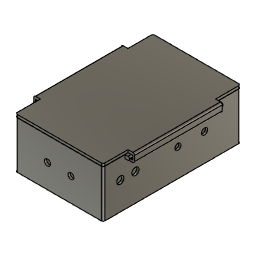
candlestick-mic (Autodesk Fusion 360 design; units mm, degrees)
Autodesk Fusion 360 part; units mm, degrees
note: some values were not read from the file. Set by a fixed rule: which sketch regions a step uses.
sketch "top" plane through (0, 0, 0) normal (0, 0, 1) x (1, 0, 0)
  line L0 (45.5, -15.075) -> (-45.5, -15.075) construction
  line L1 (-45.5, -15.075) -> (-45.5, 15.075) construction
  line L2 (-45.5, 15.075) -> (45.5, 15.075) construction
  line L3 (45.5, 15.075) -> (45.5, -15.075) construction
  line L4 (45.5, -15.075) -> (-45.5, 15.075) construction
  line L5 (-45.5, -15.075) -> (45.5, 15.075) construction
  line L6 (0, 15.075) -> (0, -15.075) construction
  line L7 (-45.5, 0) -> (45.5, 0) construction
  circle A0 centre (-40.35, 0) radius 2.1 construction
  line L8 (-35.35, 15.075) -> (-35.35, -15.075) construction
  circle A1 centre (40.35, 0) radius 2.1 construction
  line L9 (35.35, 15.075) -> (35.35, -15.075) construction
  line L10 (35.35, 33.075) -> (-4.8, 33.075) construction
  line L11 (-4.8, 33.075) -> (-4.8, 93.375) construction
  line L12 (-4.8, 93.375) -> (35.35, 93.375) construction
  line L13 (35.35, 93.375) -> (35.35, 33.075) construction
  line L14 (-45.5, 21.075) -> (-25.4, 21.075)
  line L15 (-25.4, 21.075) -> (-25.4, 101.225)
  line L16 (-25.4, 101.225) -> (-45.5, 101.225)
  line L17 (-45.5, 101.225) -> (-45.5, 21.075)
  line L18 (-4.8, 63.225) -> (35.35, 63.225) construction
  line L19 (15.275, 93.375) -> (15.275, 33.075) construction
  line L20 (-45.5, 61.15) -> (-25.4, 61.15) construction
  line L21 (-35.45, 101.225) -> (-35.45, 21.075) construction
  circle A2 centre (33.25, 35.175) radius 0.85
  circle A3 centre (33.25, 35.175) radius 2.35
  circle A4 centre (33.25, 91.275) radius 0.85
  circle A5 centre (33.25, 91.275) radius 2.35
  circle A6 centre (-2.7, 35.175) radius 0.85
  circle A7 centre (-2.7, 35.175) radius 2.35
  circle A8 centre (-2.7, 91.275) radius 2.35
  circle A9 centre (-2.7, 91.275) radius 0.85
  circle A10 centre (-27.5, 23.225) radius 0.85
  circle A11 centre (-27.5, 23.225) radius 2.1
  circle A12 centre (-27.5, 99.075) radius 0.85
  circle A13 centre (-27.5, 99.075) radius 2.1
  circle A14 centre (-43.4, 23.225) radius 0.85
  circle A15 centre (-43.4, 23.225) radius 2.1
  circle A16 centre (-43.4, 99.075) radius 0.85
  circle A17 centre (-43.4, 99.075) radius 2.1
  line L22 (-47.5, 101.725) -> (47.5, 101.725)
  line L23 (47.5, 101.725) -> (47.5, -50.075)
  line L24 (47.5, -50.075) -> (-47.5, -50.075)
  line L25 (-47.5, -50.075) -> (-47.5, 101.725)
  line L26 (-39.75, 101.225) -> (-29.75, 101.225)
  line L27 (-29.75, 101.225) -> (-29.75, 102.475)
  line L28 (-29.75, 102.475) -> (-39.75, 102.475)
  line L29 (-39.75, 102.475) -> (-39.75, 101.225)
  line L30 (-34.75, 102.475) -> (-34.75, 101.225) construction
  circle A18 centre (-40.35, 0) radius 1.75
  circle A19 centre (40.35, 0) radius 1.75
  line L31 (-50, -52.575) -> (-50, 104.225)
  line L32 (-50, 104.225) -> (50, 104.225)
  line L33 (50, 104.225) -> (50, -52.575)
  line L34 (50, -52.575) -> (-50, -52.575)
  circle A20 centre (-42.5, 76.725) radius 2.5
  dimension "d1" = 91
  dimension "d2" = 30.15
  dimension "d3" = 4.2
  dimension "d4" = 10.15
  dimension "d5" = 3.05
  dimension "d6" = 40.15
  dimension "d7" = 60.3
  dimension "d8" = 18
  dimension "d9" = 20.1
  dimension "d10" = 80.15
  dimension "d11" = 6
  dimension "d12" = 1.7
  dimension "d13" = 1.25
  dimension "d14" = 1.25
  dimension "d15" = 1.5
  dimension "d16" = 1.7
  dimension "d17" = 1.25
  dimension "d18" = 1.3
  dimension "d19" = 1.25
  dimension "d20" = 2
  dimension "d21" = 1.25
  dimension "d22" = 10
  dimension "d23" = 0.5
  dimension "d24" = 2
  dimension "d25" = 35
  dimension "d35" = -0.35
  dimension "d39" = -2.5
  dimension "d43" = 4.35
  dimension "d61" = 5
  dimension "d62" = 22
  dimension "d63" = 0.5
  constraint horizontal L0
  constraint perpendicular L0 L1
  constraint parallel L0 L2
  constraint parallel L1 L3
  constraint coincident L4 origin
  constraint coincident L5 origin
  constraint midpoint L2 L6.start
  constraint midpoint L0 L6.end
  constraint midpoint L1 L7.start
  constraint midpoint L3 L7.end
  constraint coincident L7 A0.centre
  constraint coincident L2 L8.start
  constraint coincident L0 L8.end
  constraint perpendicular L0 L8
  constraint symmetric L6 A0 A1
  constraint symmetric L6 L8.start L9.start
  constraint symmetric L6 L8.end L9.end
  constraint horizontal L10
  constraint vertical L11
  constraint horizontal L12
  constraint vertical L13
  constraint horizontal L14
  constraint vertical L15
  constraint horizontal L16
  constraint vertical L17
  constraint collinear L1 L17
  constraint collinear L9 L13
  constraint midpoint L11 L18.start
  constraint midpoint L13 L18.end
  constraint midpoint L12 L19.start
  constraint midpoint L10 L19.end
  constraint midpoint L17 L20.start
  constraint midpoint L15 L20.end
  constraint midpoint L16 L21.start
  constraint midpoint L14 L21.end
  constraint symmetric L18 A2 A4
  constraint symmetric L18 A3 A5
  constraint symmetric L19 A2 A6
  constraint symmetric L19 A3 A7
  constraint symmetric L19 A4 A9
  constraint symmetric L19 A5 A8
  constraint symmetric L20 A10 A12
  constraint symmetric L20 A11 A13
  constraint symmetric L21 A10 A14
  constraint symmetric L21 A11 A15
  constraint symmetric L21 A12 A16
  constraint symmetric L21 A13 A17
  constraint horizontal L22
  constraint vertical L23
  constraint horizontal L24
  constraint vertical L25
  constraint horizontal L26
  constraint vertical L27
  constraint horizontal L28
  constraint vertical L29
  constraint coincident L16 L26.start
  constraint midpoint L28 L30.start
  constraint midpoint L26 L30.end
  constraint symmetric L6 A18 A19
  measures "d1" distance of L1.end L2.end
  measures "d2" distance of L0.end L1.end
  measures "d3" diameter of A0
  measures "d4" distance of L1 L8
  measures "d5" distance of L1 A0
  measures "d6" distance of L10.start L10.end
  measures "d7" distance of L10.start L12.end
  measures "d8" distance of L2 L10
  measures "d9" distance of L14.start L14.end
  measures "d10" distance of L14.start L16.end
  measures "d11" distance of L2 L14
  measures "d12" diameter of A2
  measures "d13" distance of L13 A2
  measures "d14" distance of L10 A2
  measures "d16" diameter of A10
  measures "d17" distance of L15 A10
  measures "d18" distance of L14 A10
  measures "d20" distance of L17 L25
  measures "d21" distance of L26.end L27.end
  measures "d22" distance of L27.end L28.end
  measures "d23" distance of L16 L22
  measures "d24" distance of L3 L23
  measures "d25" distance of L0 L24
  measures "d43" distance of L15 L27
  measures "d61" diameter of A20
  measures "d62" distance of L16 A20
  measures "d63" distance of L17 A20
extrude "Extrude1" add sketch "top" along normal blind 9 contours A11 | A13 | A17 | A15 | L14 L15 L16 L17 L26 | L14 L15 L16 L17 L22 L23 L24 L25 L27 L29 | L16 L22 L26 L27 L29 | L22 L27 L28 L29 | A2 | A3 | A4 | A5 | A6 | A7 | A8 | A9 | A10 | A12 | A14 | A16 | A18 | A19 | L31 L32 L33 L34 | A20 makes body 1
extrude "Extrude2" add sketch "top" along normal blind 12 from surface at 9 contours A11 | A13 | A17 | A15 | A3 | A5 | A7 | A8 bodies 1
extrude "Extrude4" cut sketch "top" against normal blind 6.5 from surface at 9 contours A18 | A19 bodies 1
extrude "Extrude5" add sketch "top" along normal blind 45 from surface at 9 contours L22 L27 L28 L29 | L31 L32 L33 L34 bodies 1
sketch "outputs" plane through (47.5, 0, 0) normal (-1, 0, 0) x (0, -1, 0)
  line L0 (-101.725, 9) -> (50.075, 9)
  line L1 (50.075, 9) -> (50.075, 54)
  line L2 (50.075, 54) -> (-101.725, 54)
  line L3 (-101.725, 54) -> (-101.725, 9)
  line L4 (-32.825, 21) -> (-37.525, 21)
  line L5 (-88.925, 21) -> (-93.625, 21)
  line L6 (-93.625, 21) -> (-93.625, 54) construction
  line L7 (-32.825, 21) -> (-32.825, 54) construction
  line L8 (-93.625, 54) -> (-32.825, 54) construction
  line L9 (-88.925, 21) -> (-37.525, 21) construction
  line L10 (-63.225, 21) -> (-63.225, 54) construction
  circle A0 centre (-63.225, 31.5) radius 3.5
  circle A1 centre (-32.825, 31.5) radius 3.5
  line L11 (50.075, 31.5) -> (-32.825, 31.5) construction
  line L12 (25.825, 24.9389) -> (25.825, 54) construction
  circle A2 centre (32.95, 31.5) radius 4.125
  circle A3 centre (15.7, 31.5) radius 4.125
  line L13 (-32.825, 31.5) -> (-63.225, 31.5) construction
  dimension "d44" = 7
  dimension "d45" = 7
  dimension "d46" = 8.25
  dimension "d47" = 8.25
  dimension "d48" = 6
  dimension "d49" = 3
  dimension "d50" = 13
  constraint coincident L5.end L6.start
  constraint coincident L2 L6.end
  constraint perpendicular L2 L6
  constraint coincident L4.start L7.start
  constraint coincident L2 L7.end
  constraint perpendicular L2 L7
  constraint coincident L5.start L9.start
  constraint coincident L4.end L9.end
  constraint midpoint L9 L10.start
  constraint midpoint L8 L10.end
  constraint midpoint L1 L11.start
  constraint coincident L7 A1.centre
  constraint perpendicular L7 L11
  constraint coincident L2 L12.end
  constraint perpendicular L2 L12
  constraint coincident L11 A2.centre
  constraint coincident L11 A3.centre
  constraint coincident A1.centre L11.end
  constraint coincident L10 A0.centre
  constraint perpendicular L10 L13
  constraint coincident A0.centre L13.end
  measures "d44" diameter of A0
  measures "d45" diameter of A1
  measures "d46" diameter of A2
  measures "d47" diameter of A3
  measures "d48" distance of L12 A3
  measures "d49" distance of L12 A2
  measures "d50" distance of L1 A2
extrude "Extrude6" cut sketch "outputs" against normal blind 4 contours A0 | A1 | A2 | A3 bodies 1
extrude "Extrude7" add sketch "top" along normal blind 1.5 from surface at 21 separate body contours A11 | A13 | A17 | A15 | L14 L15 L16 L17 L26 | A10 | A12 | A14 | A16 | A20 makes body 2
extrude "Extrude8" add sketch "top" along normal blind 12 from surface at 22.5 contours L16 L22 L26 L27 L29 | L22 L27 L28 L29 bodies 2
extrude "Extrude9" cut 1 faces at (-33.0833, 102.475, 26.5) along direction (0, 1, 0) blind 5 on bodies 2 bodies 1
extrude "Extrude10" add sketch "top" along normal blind 7 from surface at 22.5 contours A20 bodies 2
sketch "side" plane through (-47.5, 0, 0) normal (1, 0, 0) x (0, 1, 0)
  line L0 (-50.075, 9) -> (101.725, 9)
  line L1 (101.725, 9) -> (101.725, 54)
  line L2 (101.725, 54) -> (-50.075, 54)
  line L3 (-50.075, 54) -> (-50.075, 9)
  line L4 (79.225, 29.5) -> (74.225, 29.5)
  line L5 (74.225, 22.5) -> (79.225, 22.5)
  line L6 (76.725, 29.5) -> (76.725, 22.5) construction
  line L7 (74.225, 29.5) -> (74.225, 22.5) construction
  line L8 (79.225, 29.5) -> (79.225, 22.5) construction
  line L9 (74.225, 26) -> (79.225, 26) construction
  line L10 (74.975, 27.75) -> (78.475, 27.75)
  line L11 (78.475, 27.75) -> (78.475, 24.25)
  line L12 (78.475, 24.25) -> (74.975, 24.25)
  line L13 (74.975, 24.25) -> (74.975, 27.75)
  line L14 (74.975, 26) -> (78.475, 26) construction
  line L15 (76.725, 27.75) -> (76.725, 24.25) construction
  point P0 (76.725, 26)
  point P1 (76.725, 26)
  dimension "d67" = 3.5
  dimension "d68" = 3.5
  constraint midpoint L4 L6.start
  constraint midpoint L5 L6.end
  constraint coincident L4.end L7.start
  constraint coincident L5.start L7.end
  constraint coincident L4.start L8.start
  constraint coincident L5.end L8.end
  constraint midpoint L7 L9.start
  constraint midpoint L8 L9.end
  constraint horizontal L10
  constraint vertical L11
  constraint horizontal L12
  constraint vertical L13
  constraint midpoint L6 P1
  constraint midpoint L13 L14.start
  constraint midpoint L11 L14.end
  constraint midpoint L10 L15.start
  constraint midpoint L12 L15.end
  constraint midpoint L14 P1
  constraint coincident P1 P0
  measures "d67" distance of L10.start L10.end
  measures "d68" distance of L10.start L12.end
extrude "Extrude11" cut sketch "side" against normal blind 5 contours L10 L11 L12 L13 bodies 1
extrude "Extrude12" cut 1 faces at (-33.0833, 102.475, 26.5) along direction (0, -1, 0) blind 1 on bodies 1 bodies 1
sketch "inputs" plane through (0, -52.575, 0) normal (0, -1, 0) x (1, 0, 0)
  line L0 (-50, 0) -> (50, 0)
  line L1 (50, 0) -> (50, 54)
  line L2 (50, 54) -> (-50, 54)
  line L3 (-50, 54) -> (-50, 0)
  line L4 (47.5, 9) -> (-47.5, 9)
  line L5 (-47.5, 9) -> (-47.5, 54)
  line L6 (-47.5, 54) -> (47.5, 54)
  line L7 (47.5, 54) -> (47.5, 9)
  line L8 (0, 54) -> (0, 9) construction
  line L9 (47.5, 31.5) -> (-47.5, 31.5) construction
  circle A0 centre (13.375, 27) radius 3.375
  circle A1 centre (-13.5, 27) radius 3.5
  line L10 (50, 0) -> (-50, 0)
  line L11 (-35.6219, 54) -> (-35.6219, 0) construction
  line L12 (-35.6219, 27) -> (47.5, 27) construction
  dimension "d73" = 6.75
  dimension "d74" = 7
  dimension "d75" = 10
  dimension "d76" = 10
  constraint midpoint L6 L8.start
  constraint midpoint L4 L8.end
  constraint midpoint L7 L9.start
  constraint midpoint L5 L9.end
  constraint coincident L2 L11.start
  constraint coincident L10 L11.end
  constraint perpendicular L10 L11
  constraint midpoint L11 L12.start
  constraint coincident L7 L12.end
  constraint perpendicular L7 L12
  constraint coincident A1.centre L12
  constraint coincident A0.centre L12
  measures "d73" diameter of A0
  measures "d74" diameter of A1
  measures "d75" distance of L8 A0
  measures "d76" distance of L8 A1
extrude "Extrude13" cut sketch "inputs" against normal blind 4 contours A0 | A1 bodies 1
sketch "lid_bottom" plane through (-50, 0, 0) normal (-1, 0, 0) x (0, -1, 0)
  line L0 (-78.475, 24.25) -> (-78.475, 27.75)
  line L1 (-78.475, 27.75) -> (-74.975, 27.75)
  line L2 (-74.975, 27.75) -> (-74.975, 24.25)
  line L3 (-74.975, 24.25) -> (-78.475, 24.25)
  line L4 (-104.225, 0) -> (52.575, 0)
  line L5 (52.575, 0) -> (52.575, 54)
  line L6 (52.575, 54) -> (-104.225, 54)
  line L7 (-104.225, 54) -> (-104.225, 0)
  line L8 (-104.225, 54) -> (52.575, 54)
  line L9 (-104.225, 0) -> (-104.225, 54)
  line L10 (52.575, 0) -> (-104.225, 0)
  line L11 (52.575, 0) -> (52.575, 54)
  line L12 (-25.825, 54) -> (-25.825, 0) construction
  line L13 (-25.825, 50) -> (27.575, 50)
  line L14 (27.575, 50) -> (27.575, 54)
  line L15 (-25.825, 50) -> (-79.225, 50)
  line L16 (-79.225, 50) -> (-79.225, 54)
  dimension "d79" = 25
  dimension "d80" = 4
  constraint midpoint L8 L12.start
  constraint midpoint L10 L12.end
  constraint coincident L12 L13.start
  constraint perpendicular L12 L13
  constraint coincident L8 L14.end
  constraint perpendicular L8 L14
  constraint symmetric L12 L13.start L15.start
  constraint symmetric L12 L13.end L15.end
  constraint symmetric L12 L14.end L16.end
  measures "d79" distance of L11 L14
  measures "d80" distance of L8 L13
extrude "Extrude14" add sketch "lid_bottom" along normal blind 5 contours L6 L8 L13 L14 L15 L16 bodies 1
extrude "Extrude15" add sketch "lid_bottom" against normal blind 5 from surface at -100 contours L6 L8 L13 L14 L15 L16 bodies 1
fillet "Fillet1" radius 1.5 4 edges at (-55, 25.825, 54) (-55, 25.825, 50) (55, 25.825, 54) (55, 25.825, 50) on bodies 1
sketch "lid_top" plane through (0, 104.225, 0) normal (0, 1, 0) x (-1, 0, 0)
  line L0 (29.75, 22.5) -> (29.75, 34.5)
  line L1 (29.75, 34.5) -> (39.75, 34.5)
  line L2 (39.75, 34.5) -> (39.75, 22.5)
  line L3 (39.75, 22.5) -> (29.75, 22.5)
  line L4 (-50, 0) -> (50, 0)
  line L5 (50, 0) -> (50, 54)
  line L6 (50, 54) -> (-50, 54)
  line L7 (-50, 54) -> (-50, 0)
  line L8 (50, 54) -> (53.5, 54)
  arc A0 (55, 52.5) -> (53.5, 54) centre (53.5, 52.5) ccw
  line L9 (55, 52.5) -> (55, 51.5)
  arc A1 (53.5, 50) -> (55, 51.5) centre (53.5, 51.5) ccw
  line L10 (50, 50) -> (53.5, 50)
  line L11 (50, 50) -> (50, 54)
  line L12 (-50, 54) -> (-53.5, 54)
  arc A2 (-53.5, 54) -> (-55, 52.5) centre (-53.5, 52.5) ccw
  arc A3 (-55, 51.5) -> (-53.5, 50) centre (-53.5, 51.5) ccw
  line L13 (-50, 50) -> (-53.5, 50)
  line L14 (-50, 54) -> (-50, 50)
  line L15 (-55, 51.5) -> (-55, 52.5)
  line L16 (-50, 54) -> (50, 54)
  line L17 (-55, 52) -> (-57.5, 52) construction
  line L18 (-51, 49.75) -> (-51, 47.25)
  line L19 (-57.5, 52) -> (-57.5, 57.25)
  line L20 (-57.5, 52) -> (-57.5, 47.25)
  line L21 (-57.5, 47.25) -> (-51, 47.25)
  line L22 (0, 54) -> (0, 70) construction
  line L23 (0, 54) -> (0, 39) construction
  line L24 (-55, 49.75) -> (-55, 54.25)
  line L25 (-57.5, 57.25) -> (0, 57.25)
  line L26 (-55, 54.25) -> (0, 54.25)
  line L27 (-55, 49.75) -> (-51, 49.75)
  line L28 (57.5, 57.25) -> (0, 57.25)
  line L29 (55, 54.25) -> (0, 54.25)
  line L30 (57.5, 52) -> (57.5, 57.25)
  line L31 (55, 49.75) -> (55, 54.25)
  line L32 (57.5, 52) -> (57.5, 47.25)
  line L33 (57.5, 47.25) -> (51, 47.25)
  line L34 (51, 49.75) -> (51, 47.25)
  line L35 (55, 49.75) -> (51, 49.75)
  line L36 (50, 57.25) -> (50, 54.25)
  line L37 (-50, 57.25) -> (-50, 54.25)
  line L38 (45.5, 21) -> (41.3, 21)
  line L39 (29.6, 21) -> (25.4, 21)
  line L40 (5.05, 21) -> (0.35, 21)
  line L41 (-30.9, 21) -> (-35.6, 21)
  line L42 (5.05, 21) -> (25.4, 21) construction
  line L43 (39.75, 22.5) -> (39.75, 34.5)
  line L44 (39.75, 34.5) -> (29.75, 34.5)
  line L45 (29.75, 34.5) -> (29.75, 22.5)
  line L46 (29.75, 22.5) -> (39.75, 22.5)
  line L47 (29.75, 28.5) -> (0, 28.5) construction
  line L48 (15.225, 21) -> (15.225, 28.5) construction
  circle A4 centre (15.225, 28.5) radius 3
  dimension "d88" = 2.5
  dimension "d90" = 2.5
  dimension "d91" = 2.5
  dimension "d92" = 1
  dimension "d94" = 0.25
  dimension "d95" = 3
  dimension "d96" = 4.5
  dimension "d108" = 7.5
  dimension "d119" = 6
  constraint midpoint L15 L17.start
  constraint perpendicular L15 L17
  constraint perpendicular L13 L18
  constraint perpendicular L17 L19
  constraint perpendicular L17 L20
  constraint perpendicular L20 L21
  constraint midpoint L6 L22.start
  constraint perpendicular L16 L22
  constraint perpendicular L16 L23
  constraint perpendicular L17 L24
  constraint coincident L22 L25.end
  constraint perpendicular L22 L25
  constraint coincident L22 L26.end
  constraint perpendicular L22 L26
  constraint perpendicular L18 L27
  constraint symmetric L17.end L23 L30.start
  constraint symmetric L18.start L23 L34.start
  constraint symmetric L18.end L23 L33.end
  constraint symmetric L19.end L23 L28.start
  constraint symmetric L20.end L23 L32.end
  constraint symmetric L23 L24.start L31.start
  constraint symmetric L23 L25.end L28.end
  constraint symmetric L23 L24.end L29.start
  constraint symmetric L23 L26.end L29.end
  constraint coincident L28 L36.start
  constraint coincident L29 L36.end
  constraint perpendicular L29 L36
  constraint symmetric L22 L36.start L37.start
  constraint symmetric L22 L36.end L37.end
  constraint coincident L40.start L42.start
  constraint coincident L39.end L42.end
  constraint midpoint L45 L47.start
  constraint perpendicular L45 L47
  constraint midpoint L42 L48.start
  constraint coincident L47 L48.end
  constraint perpendicular L47 L48
  constraint coincident L48.end A4.centre
  measures "d88" distance of L17.start L17.end
  measures "d90" distance of L18.start L18.end
  measures "d91" distance of L19 L24
  measures "d92" distance of L7 L18
  measures "d94" distance of L16 L26
  measures "d95" distance of L25 L26
  measures "d96" distance of L24.start L24.end
  measures "d108" distance of L30 L36
  measures "d119" diameter of A4
ref_plane "WorkPlane1" through (0, 25.825, 27) normal (0, -1, 0) x (1, 0, 0)
extrude "Extrude17" add sketch "lid_top" along normal blind 50 and the other way blind 50 from surface at -78.4 separate body contours L15 L18 L19 L20 L21 L24 L25 L26 L27 L37 | L9 L28 L29 L30 L31 L32 L33 L34 L35 L36 | L25 L26 L28 L29 L36 L37 makes body 3
extrude "Extrude18" add sketch "lid_top" against normal up to surface (28.4 mm away) from surface at -128.4 contours L25 L26 L28 L29 L36 L37 bodies 3
extrude "Extrude19" add sketch "lid_top" along normal up to surface (28.4 mm away) from surface at -28.4 contours L25 L26 L28 L29 L36 L37 bodies 3
fillet "Fillet4" radius 2 4 edges at (57.5, 25.825, 57.25) (57.5, 25.825, 47.25) (-57.5, 25.825, 47.25) (-57.5, 25.825, 57.25) on bodies 3
fillet "Fillet5" radius 2 8 edges at (50, 104.225, 27) (-50, 104.225, 27) (-50, -52.575, 27) (50, -52.575, 27) (50, 104.225, 55.75) (-50, 104.225, 55.75) (-50, -52.575, 55.75) (50, -52.575, 55.75) on bodies 1 3
extrude "Extrude20" cut sketch "lid_top" against normal blind 4 contours A4 bodies 1
move_face "OffsetFaces1" offset -0.5 1 faces at (55, 9.1583, 51.25) on bodies 3
move_face "OffsetFaces2" offset -0.5 1 faces at (-55, 9.1583, 51.25) on bodies 3
hidden bodies 2
named bodies: "enclosure", "board_psu", "lid"
